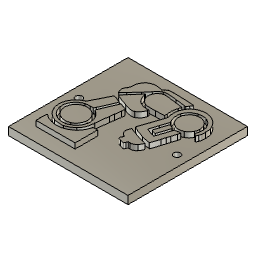
logo positive (Autodesk Fusion 360 design; units mm, degrees)
Autodesk Fusion 360 part; units mm, degrees
sketch "Sketch1" plane through (0, 0, 0) normal (0, 0, 1) x (1, 0, 0)
  line L0 (0, 0) -> (45, 0)
  line L1 (45, 0) -> (45, 45)
  line L2 (45, 45) -> (0, 45)
  line L3 (0, 45) -> (0, 0)
  dimension "d1" = 45
  dimension "d2" = 45
  constraint horizontal L0
  constraint vertical L1
  constraint horizontal L2
  constraint vertical L3
  constraint coincident L0.start L3.end
  measures "d1" distance of L0.start L0.end
  measures "d2" distance of L0.start L2.end
extrude "Extrude1" add sketch "Sketch1" along normal blind 3
sketch "Sketch2" plane through (0, 0, 3) normal (0, 0, 1) x (-1, 0, 0)
  line L0 (0, -45) -> (0, 0)
  line L1 (0, 0) -> (-45, 0)
  line L2 (-45, 0) -> (-45, -45)
  line L3 (-45, -45) -> (0, -45)
  spline S0 degree 3 poles (-20.2484, -39.8736) (-20.0856, -39.7573) (-19.7484, -39.4783) (-19.481, -39.2225) knots 0 0 0 0 1 1 1 1
  line L4 (-19.481, -39.2225) -> (-19.0044, -38.7691)
  line L5 (-19.0044, -38.7691) -> (-18.0859, -38.9668)
  spline S1 degree 3 poles (-18.0859, -38.9668) (-16.8071, -39.2342) (-15.5166, -39.1528) (-14.6447, -38.7575) knots 0 0 0 0 1 1 1 1
  spline S2 degree 3 poles (-14.6447, -38.7575) (-13.0519, -38.0251) (-12.1218, -36.3975) (-12.1102, -34.3164) knots 0 0 0 0 1 1 1 1
  spline S3 degree 3 poles (-12.1102, -34.3164) (-12.0986, -33.8281) (-12.0288, -33.6072) (-11.6452, -33.0376) knots 0 0 0 0 1 1 1 1
  spline S4 degree 3 poles (-11.6452, -33.0376) (-11.1685, -32.3168) (-10.9825, -31.6076) (-11.1104, -30.9798) knots 0 0 0 0 1 1 1 1
  spline S5 degree 3 poles (-11.1104, -30.9798) (-11.1918, -30.5264) (-11.5289, -29.8288) (-11.6452, -29.8288) knots 0 0 0 0 1 1 1 1
  spline S6 degree 3 poles (-11.6452, -29.8288) (-11.7033, -29.8288) (-12.3892, -30.5147) (-13.1798, -31.3634) knots 0 0 0 0 1 1 1 1
  spline S7 degree 3 poles (-13.1798, -31.3634) (-13.9704, -32.2005) (-15.1795, -33.491) (-15.8654, -34.2234) knots 0 0 0 0 1 1 1 1
  spline S8 degree 3 poles (-15.8654, -34.2234) (-16.5629, -34.9558) (-17.4116, -35.9324) (-17.7488, -36.3975) knots 0 0 0 0 1 1 1 1
  spline S9 degree 3 poles (-17.7488, -36.3975) (-18.4463, -37.3392) (-19.2369, -38.0716) (-19.8763, -38.3855) knots 0 0 0 0 1 1 1 1
  spline S10 degree 3 poles (-19.8763, -38.3855) (-20.5739, -38.7226) (-21.6086, -38.711) (-24.7825, -38.3274) knots 0 0 0 0 1 1 1 1
  spline S11 degree 3 poles (-24.7825, -38.3274) (-26.4101, -38.1297) (-28.0144, -37.9321) (-28.3283, -37.8972) knots 0 0 0 0 1 1 1 1
  line L6 (-28.3283, -37.8972) -> (-28.9096, -37.8391)
  line L7 (-28.9096, -37.8391) -> (-29.5142, -38.7459)
  spline S12 degree 3 poles (-29.5142, -38.7459) (-30.0374, -39.5248) (-30.0955, -39.6643) (-29.9211, -39.7225) knots 0 0 0 0 1 1 1 1
  spline S13 degree 3 poles (-29.9211, -39.7225) (-29.6421, -39.8271) (-24.3639, -40.0596) (-22.2713, -40.0596) knots 0 0 0 0 1 1 1 1
  spline S14 degree 3 poles (-22.2713, -40.0596) (-20.8529, -40.0596) (-20.4809, -40.0247) (-20.2484, -39.8736) knots 0 0 0 0 1 1 1 1
  spline S15 degree 3 poles (-33.0368, -39.3272) (-31.9789, -39.0133) (-30.8628, -38.3506) (-30.3164, -37.7228) knots 0 0 0 0 1 1 1 1
  spline S16 degree 3 poles (-30.3164, -37.7228) (-29.7816, -37.0834) (-29.1305, -35.8278) (-28.9096, -34.9907) knots 0 0 0 0 1 1 1 1
  spline S17 degree 3 poles (-28.9096, -34.9907) (-28.712, -34.235) (-28.6888, -32.712) (-28.8631, -31.9215) knots 0 0 0 0 1 1 1 1
  spline S18 degree 3 poles (-28.8631, -31.9215) (-29.084, -30.91) (-29.1073, -30.5264) (-28.991, -30.3869) knots 0 0 0 0 1 1 1 1
  spline S19 degree 3 poles (-28.991, -30.3869) (-28.9329, -30.3055) (-28.8166, -30.0497) (-28.7585, -29.8288) knots 0 0 0 0 1 1 1 1
  spline S20 degree 3 poles (-28.7585, -29.8288) (-28.6888, -29.6079) (-28.1075, -27.8757) (-27.4564, -25.9923) knots 0 0 0 0 1 1 1 1
  spline S21 degree 3 poles (-27.4564, -25.9923) (-26.2008, -22.3534) (-26.0264, -21.7953) (-26.0846, -21.7604) knots 0 0 0 0 1 1 1 1
  spline S22 degree 3 poles (-26.0846, -21.7604) (-26.724, -21.2954) (-28.8864, -20.4002) (-30.4908, -19.9352) knots 0 0 0 0 1 1 1 1
  spline S23 degree 3 poles (-30.4908, -19.9352) (-31.8742, -19.5399) (-33.56, -19.2028) (-33.7576, -19.2841) knots 0 0 0 0 1 1 1 1
  spline S24 degree 3 poles (-33.7576, -19.2841) (-33.9088, -19.3423) (-34.1413, -19.9701) (-34.897, -22.5045) knots 0 0 0 0 1 1 1 1
  spline S25 degree 3 poles (-34.897, -22.5045) (-35.0946, -23.1788) (-35.3039, -23.8531) (-35.362, -24.0159) knots 0 0 0 0 1 1 1 1
  spline S26 degree 3 poles (-35.362, -24.0159) (-35.4201, -24.1786) (-35.5945, -24.7832) (-35.7689, -25.3529) knots 0 0 0 0 1 1 1 1
  spline S27 degree 3 poles (-35.7689, -25.3529) (-35.9433, -25.9341) (-36.2107, -26.8061) (-36.3735, -27.3176) knots 0 0 0 0 1 1 1 1
  spline S28 degree 3 poles (-36.3735, -27.3176) (-36.5246, -27.8175) (-36.6292, -28.2477) (-36.606, -28.2826) knots 0 0 0 0 1 1 1 1
  spline S29 degree 3 poles (-36.606, -28.2826) (-36.5711, -28.3058) (-36.0828, -28.271) (-35.5015, -28.1896) knots 0 0 0 0 1 1 1 1
  line L8 (-35.5015, -28.1896) -> (-34.4552, -28.0617)
  line L9 (-34.4552, -28.0617) -> (-33.5135, -25.1668)
  spline S30 degree 3 poles (-33.5135, -25.1668) (-32.9903, -23.5857) (-32.5253, -22.2604) (-32.4788, -22.2255) knots 0 0 0 0 1 1 1 1
  spline S31 degree 3 poles (-32.4788, -22.2255) (-32.3625, -22.1557) (-29.3282, -23.1439) (-29.177, -23.2951) knots 0 0 0 0 1 1 1 1
  spline S32 degree 3 poles (-29.177, -23.2951) (-29.0957, -23.3764) (-29.4444, -24.5855) (-30.1187, -26.6084) knots 0 0 0 0 1 1 1 1
  line L10 (-30.1187, -26.6084) -> (-31.1767, -29.8056)
  line L11 (-31.1767, -29.8056) -> (-30.886, -30.3055)
  spline S33 degree 3 poles (-30.886, -30.3055) (-30.1769, -31.5495) (-29.9327, -33.305) (-30.3048, -34.5489) knots 0 0 0 0 1 1 1 1
  spline S34 degree 3 poles (-30.3048, -34.5489) (-30.7117, -35.9208) (-32.1533, -37.2926) (-33.6414, -37.7461) knots 0 0 0 0 1 1 1 1
  spline S35 degree 3 poles (-33.6414, -37.7461) (-34.5133, -38.0135) (-35.7805, -38.0135) (-36.6641, -37.7461) knots 0 0 0 0 1 1 1 1
  spline S36 degree 3 poles (-36.6641, -37.7461) (-37.8267, -37.3857) (-39.0707, -36.1766) (-39.5822, -34.9093) knots 0 0 0 0 1 1 1 1
  spline S37 degree 3 poles (-39.5822, -34.9093) (-39.8961, -34.142) (-39.9194, -32.3633) (-39.6171, -31.5843) knots 0 0 0 0 1 1 1 1
  spline S38 degree 3 poles (-39.6171, -31.5843) (-39.3264, -30.8054) (-39.373, -30.5961) (-39.838, -30.3752) knots 0 0 0 0 1 1 1 1
  spline S39 degree 3 poles (-39.838, -30.3752) (-40.0705, -30.2706) (-40.2681, -30.1776) (-40.2914, -30.1776) knots 0 0 0 0 1 1 1 1
  spline S40 degree 3 poles (-40.2914, -30.1776) (-40.3146, -30.1776) (-40.489, -30.5264) (-40.6634, -30.9682) knots 0 0 0 0 1 1 1 1
  spline S41 degree 3 poles (-40.6634, -30.9682) (-40.9773, -31.689) (-41.0006, -31.8517) (-40.989, -33.2003) knots 0 0 0 0 1 1 1 1
  spline S42 degree 3 poles (-40.989, -33.2003) (-40.9773, -34.4443) (-40.9308, -34.7698) (-40.6983, -35.4093) knots 0 0 0 0 1 1 1 1
  spline S43 degree 3 poles (-40.6983, -35.4093) (-39.5125, -38.5715) (-36.2107, -40.2573) (-33.0368, -39.3272) knots 0 0 0 0 1 1 1 1
  spline S44 degree 3 poles (-20.6088, -37.5949) (-20.0042, -37.4322) (-19.2485, -36.8625) (-18.8649, -36.2928) knots 0 0 0 0 1 1 1 1
  spline S45 degree 3 poles (-18.8649, -36.2928) (-17.6093, -34.4676) (-18.5045, -31.8168) (-20.6669, -30.9914) knots 0 0 0 0 1 1 1 1
  spline S46 degree 3 poles (-20.6669, -30.9914) (-21.3412, -30.7356) (-21.4226, -30.7356) (-24.5383, -30.8054) knots 0 0 0 0 1 1 1 1
  spline S47 degree 3 poles (-24.5383, -30.8054) (-26.2938, -30.8403) (-27.7819, -30.9217) (-27.8401, -30.9798) knots 0 0 0 0 1 1 1 1
  spline S48 degree 3 poles (-27.8401, -30.9798) (-27.8982, -31.0379) (-27.8866, -31.4448) (-27.7936, -31.968) knots 0 0 0 0 1 1 1 1
  spline S49 degree 3 poles (-27.7936, -31.968) (-27.6075, -33.1771) (-27.7238, -34.6303) (-28.1075, -35.8394) knots 0 0 0 0 1 1 1 1
  spline S50 degree 3 poles (-28.1075, -35.8394) (-28.2818, -36.3742) (-28.3981, -36.8276) (-28.3749, -36.8509) knots 0 0 0 0 1 1 1 1
  spline S51 degree 3 poles (-28.3749, -36.8509) (-28.2935, -36.9322) (-21.8411, -37.7344) (-21.4109, -37.7228) knots 0 0 0 0 1 1 1 1
  spline S52 degree 3 poles (-21.4109, -37.7228) (-21.19, -37.7228) (-20.8296, -37.6647) (-20.6088, -37.5949) knots 0 0 0 0 1 1 1 1
  spline S53 degree 3 poles (-34.1297, -36.9322) (-33.0136, -36.6648) (-31.9905, -35.851) (-31.4325, -34.7698) knots 0 0 0 0 1 1 1 1
  spline S54 degree 3 poles (-31.4325, -34.7698) (-31.1534, -34.2583) (-31.1186, -34.0606) (-31.1186, -33.0259) knots 0 0 0 0 1 1 1 1
  spline S55 degree 3 poles (-31.1186, -33.0259) (-31.1186, -31.9796) (-31.1534, -31.8052) (-31.4441, -31.2472) knots 0 0 0 0 1 1 1 1
  spline S56 degree 3 poles (-31.4441, -31.2472) (-32.4672, -29.3057) (-34.7458, -28.5383) (-36.699, -29.48) knots 0 0 0 0 1 1 1 1
  spline S57 degree 3 poles (-36.699, -29.48) (-37.3849, -29.8172) (-38.1987, -30.6543) (-38.5824, -31.4332) knots 0 0 0 0 1 1 1 1
  spline S58 degree 3 poles (-38.5824, -31.4332) (-38.8614, -32.0145) (-38.9079, -32.2354) (-38.9079, -33.1422) knots 0 0 0 0 1 1 1 1
  spline S59 degree 3 poles (-38.9079, -33.1422) (-38.9079, -34.0723) (-38.873, -34.2699) (-38.5591, -34.8628) knots 0 0 0 0 1 1 1 1
  spline S60 degree 3 poles (-38.5591, -34.8628) (-37.7453, -36.4788) (-35.8736, -37.3392) (-34.1297, -36.9322) knots 0 0 0 0 1 1 1 1
  spline S61 degree 3 poles (-16.5281, -33.6189) (-16.1793, -33.212) (-15.2957, -32.2005) (-14.5633, -31.3867) knots 0 0 0 0 1 1 1 1
  spline S62 degree 3 poles (-14.5633, -31.3867) (-12.8427, -29.4335) (-12.5404, -29.0266) (-12.7031, -28.829) knots 0 0 0 0 1 1 1 1
  spline S63 degree 3 poles (-12.7031, -28.829) (-12.8659, -28.6314) (-14.6912, -27.9222) (-16.9931, -27.1549) knots 0 0 0 0 1 1 1 1
  spline S64 degree 3 poles (-16.9931, -27.1549) (-19.1904, -26.4224) (-20.1088, -26.3062) (-20.8529, -26.6782) knots 0 0 0 0 1 1 1 1
  spline S65 degree 3 poles (-20.8529, -26.6782) (-21.876, -27.1665) (-22.7712, -28.3291) (-22.9688, -29.4103) knots 0 0 0 0 1 1 1 1
  line L12 (-22.9688, -29.4103) -> (-23.0502, -29.8637)
  line L13 (-23.0502, -29.8637) -> (-22.3875, -29.7939)
  spline S66 degree 3 poles (-22.3875, -29.7939) (-21.0505, -29.6544) (-19.7368, -30.1311) (-18.7254, -31.1193) knots 0 0 0 0 1 1 1 1
  spline S67 degree 3 poles (-18.7254, -31.1193) (-18.0627, -31.7703) (-17.4814, -32.9097) (-17.3768, -33.7933) knots 0 0 0 0 1 1 1 1
  spline S68 degree 3 poles (-17.3768, -33.7933) (-17.3419, -34.1072) (-17.2721, -34.3629) (-17.2372, -34.3513) knots 0 0 0 0 1 1 1 1
  spline S69 degree 3 poles (-17.2372, -34.3513) (-17.2024, -34.3513) (-16.8768, -34.0141) (-16.5281, -33.6189) knots 0 0 0 0 1 1 1 1
  spline S70 degree 3 poles (-31.8394, -28.9336) (-31.665, -28.643) (-30.235, -24.0856) (-30.2699, -23.9345) knots 0 0 0 0 1 1 1 1
  spline S71 degree 3 poles (-30.2699, -23.9345) (-30.3048, -23.7485) (-31.8161, -23.2253) (-31.944, -23.3532) knots 0 0 0 0 1 1 1 1
  spline S72 degree 3 poles (-31.944, -23.3532) (-32.0138, -23.423) (-33.2694, -27.3641) (-33.4321, -28.0036) knots 0 0 0 0 1 1 1 1
  spline S73 degree 3 poles (-33.4321, -28.0036) (-33.4902, -28.271) (-33.467, -28.3407) (-33.2112, -28.4337) knots 0 0 0 0 1 1 1 1
  spline S74 degree 3 poles (-33.2112, -28.4337) (-33.0601, -28.4918) (-32.6997, -28.6546) (-32.4323, -28.7825) knots 0 0 0 0 1 1 1 1
  spline S75 degree 3 poles (-32.4323, -28.7825) (-31.8742, -29.0499) (-31.9091, -29.0383) (-31.8394, -28.9336) knots 0 0 0 0 1 1 1 1
  spline S76 degree 3 poles (-11.901, -27.8175) (-11.8312, -27.7362) (-11.0174, -26.1434) (-10.0873, -24.2833) knots 0 0 0 0 1 1 1 1
  line L14 (-10.0873, -24.2833) -> (-8.3899, -20.8769)
  line L15 (-8.3899, -20.8769) -> (-7.5994, -20.5049)
  spline S77 degree 3 poles (-7.5994, -20.5049) (-6.5065, -19.9701) (-5.3207, -18.7726) (-4.751, -17.6216) knots 0 0 0 0 1 1 1 1
  spline S78 degree 3 poles (-4.751, -17.6216) (-4.007, -16.1103) (-3.914, -14.3896) (-4.4953, -12.7155) knots 0 0 0 0 1 1 1 1
  spline S79 degree 3 poles (-4.4953, -12.7155) (-5.0998, -10.9832) (-6.5879, -9.5533) (-8.4597, -8.8906) knots 0 0 0 0 1 1 1 1
  spline S80 degree 3 poles (-8.4597, -8.8906) (-9.3433, -8.5883) (-11.1453, -8.472) (-12.0056, -8.6697) knots 0 0 0 0 1 1 1 1
  spline S81 degree 3 poles (-12.0056, -8.6697) (-13.1914, -8.9371) (-14.3075, -9.5649) (-15.2027, -10.4601) knots 0 0 0 0 1 1 1 1
  spline S82 degree 3 poles (-15.2027, -10.4601) (-16.5164, -11.7738) (-16.9931, -12.948) (-17.1675, -15.3546) knots 0 0 0 0 1 1 1 1
  spline S83 degree 3 poles (-17.1675, -15.3546) (-17.2256, -16.2498) (-17.4814, -18.3889) (-17.7488, -20.2956) knots 0 0 0 0 1 1 1 1
  spline S84 degree 3 poles (-17.7488, -20.2956) (-17.7837, -20.5862) (-17.8883, -21.3419) (-17.9697, -21.9813) knots 0 0 0 0 1 1 1 1
  spline S85 degree 3 poles (-17.9697, -21.9813) (-18.0627, -22.6208) (-18.2022, -23.6438) (-18.2836, -24.26) knots 0 0 0 0 1 1 1 1
  spline S86 degree 3 poles (-18.2836, -24.26) (-18.365, -24.8646) (-18.3998, -25.4459) (-18.365, -25.5505) knots 0 0 0 0 1 1 1 1
  spline S87 degree 3 poles (-18.365, -25.5505) (-18.3185, -25.6551) (-17.772, -25.8993) (-17.0512, -26.1434) knots 0 0 0 0 1 1 1 1
  line L16 (-17.0512, -26.1434) -> (-15.8189, -26.5619)
  line L17 (-15.8189, -26.5619) -> (-15.6561, -26.1899)
  spline S88 degree 3 poles (-15.6561, -26.1899) (-15.4004, -25.6202) (-14.0169, -22.3766) (-13.4239, -20.935) knots 0 0 0 0 1 1 1 1
  line L18 (-13.4239, -20.935) -> (-12.8892, -19.6678)
  line L19 (-12.8892, -19.6678) -> (-13.1682, -19.4818)
  spline S89 degree 3 poles (-13.1682, -19.4818) (-15.3306, -18.0634) (-16.2258, -16.2033) (-15.8421, -13.9595) knots 0 0 0 0 1 1 1 1
  spline S90 degree 3 poles (-15.8421, -13.9595) (-15.4817, -11.8901) (-13.8192, -10.1694) (-11.7847, -9.7276) knots 0 0 0 0 1 1 1 1
  spline S91 degree 3 poles (-11.7847, -9.7276) (-8.7387, -9.0882) (-5.716, -11.1344) (-5.2509, -14.1687) knots 0 0 0 0 1 1 1 1
  spline S92 degree 3 poles (-5.2509, -14.1687) (-4.8673, -16.6799) (-6.46, -19.1446) (-8.9712, -19.8771) knots 0 0 0 0 1 1 1 1
  spline S93 degree 3 poles (-8.9712, -19.8771) (-9.413, -20.0166) (-9.9711, -20.0631) (-10.7732, -20.0514) knots 0 0 0 0 1 1 1 1
  line L20 (-10.7732, -20.0514) -> (-11.9358, -20.0166)
  line L21 (-11.9358, -20.0166) -> (-12.3079, -20.7722)
  spline S94 degree 3 poles (-12.3079, -20.7722) (-12.7496, -21.6558) (-14.9004, -26.6317) (-14.9004, -26.7828) knots 0 0 0 0 1 1 1 1
  spline S95 degree 3 poles (-14.9004, -26.7828) (-14.9004, -26.8293) (-14.5168, -27.0154) (-14.0634, -27.1781) knots 0 0 0 0 1 1 1 1
  spline S96 degree 3 poles (-14.0634, -27.1781) (-13.5983, -27.3409) (-12.9473, -27.585) (-12.6101, -27.7129) knots 0 0 0 0 1 1 1 1
  spline S97 degree 3 poles (-12.6101, -27.7129) (-12.1567, -27.8989) (-11.9823, -27.9222) (-11.901, -27.8175) knots 0 0 0 0 1 1 1 1
  spline S98 degree 3 poles (-25.7707, -20.3886) (-25.5498, -19.7957) (-25.3637, -19.0167) (-25.3637, -18.6912) knots 0 0 0 0 1 1 1 1
  spline S99 degree 3 poles (-25.3637, -18.6912) (-25.3637, -18.0518) (-25.8753, -17.1915) (-26.445, -16.9124) knots 0 0 0 0 1 1 1 1
  spline S100 degree 3 poles (-26.445, -16.9124) (-26.7123, -16.7729) (-26.9449, -16.6451) (-26.9681, -16.6334) knots 0 0 0 0 1 1 1 1
  spline S101 degree 3 poles (-26.9681, -16.6334) (-26.9797, -16.6218) (-26.8984, -16.3312) (-26.7589, -16.0056) knots 0 0 0 0 1 1 1 1
  spline S102 degree 3 poles (-26.7589, -16.0056) (-26.3752, -15.0291) (-26.3984, -15.0058) (-27.4913, -14.6687) knots 0 0 0 0 1 1 1 1
  spline S103 degree 3 poles (-27.4913, -14.6687) (-29.0027, -14.2036) (-28.9794, -14.2036) (-29.2817, -14.9477) knots 0 0 0 0 1 1 1 1
  line L22 (-29.2817, -14.9477) -> (-29.5374, -15.5871)
  line L23 (-29.5374, -15.5871) -> (-30.1769, -15.5522)
  spline S104 degree 3 poles (-30.1769, -15.5522) (-31.0372, -15.5057) (-31.7115, -15.808) (-32.2812, -16.4939) knots 0 0 0 0 1 1 1 1
  spline S105 degree 3 poles (-32.2812, -16.4939) (-32.6532, -16.9357) (-33.1531, -17.9239) (-33.1531, -18.2146) knots 0 0 0 0 1 1 1 1
  spline S106 degree 3 poles (-33.1531, -18.2146) (-33.1531, -18.2611) (-32.8043, -18.3541) (-32.3742, -18.4354) knots 0 0 0 0 1 1 1 1
  spline S107 degree 3 poles (-32.3742, -18.4354) (-31.3627, -18.6098) (-28.5027, -19.4934) (-27.096, -20.0747) knots 0 0 0 0 1 1 1 1
  spline S108 degree 3 poles (-27.096, -20.0747) (-25.852, -20.5862) (-25.8404, -20.5862) (-25.7707, -20.3886) knots 0 0 0 0 1 1 1 1
  spline S109 degree 3 poles (-9.32, -18.9586) (-7.3901, -18.4238) (-6.0183, -16.4242) (-6.2391, -14.4594) knots 0 0 0 0 1 1 1 1
  spline S110 degree 3 poles (-6.2391, -14.4594) (-6.3438, -13.5409) (-6.9716, -12.297) (-7.611, -11.7389) knots 0 0 0 0 1 1 1 1
  spline S111 degree 3 poles (-7.611, -11.7389) (-8.9131, -10.5996) (-10.936, -10.2857) (-12.4823, -10.9716) knots 0 0 0 0 1 1 1 1
  spline S112 degree 3 poles (-12.4823, -10.9716) (-15.1097, -12.1226) (-15.7259, -15.7615) (-13.6565, -17.8309) knots 0 0 0 0 1 1 1 1
  spline S113 degree 3 poles (-13.6565, -17.8309) (-12.5288, -18.9586) (-10.8779, -19.3888) (-9.32, -18.9586) knots 0 0 0 0 1 1 1 1
  spline S114 degree 3 poles (-18.2371, -13.5874) (-18.2022, -13.5293) (-18.1441, -13.3084) (-18.0976, -13.0875) knots 0 0 0 0 1 1 1 1
  spline S115 degree 3 poles (-18.0976, -13.0875) (-17.9464, -12.3435) (-17.1326, -10.8205) (-16.5048, -10.1113) knots 0 0 0 0 1 1 1 1
  spline S116 degree 3 poles (-16.5048, -10.1113) (-13.7844, -7.0188) (-9.4363, -6.5189) (-5.9485, -8.8906) knots 0 0 0 0 1 1 1 1
  line L24 (-5.9485, -8.8906) -> (-5.2858, -9.344)
  line L25 (-5.2858, -9.344) -> (-5.2044, -8.7511)
  spline S117 degree 3 poles (-5.2044, -8.7511) (-5.1696, -8.4139) (-5.1347, -7.4838) (-5.1347, -6.67) knots 0 0 0 0 1 1 1 1
  line L26 (-5.1347, -6.67) -> (-5.1347, -5.1819)
  line L27 (-5.1347, -5.1819) -> (-12.5171, -5.1819)
  line L28 (-12.5171, -5.1819) -> (-19.8996, -5.1819)
  line L29 (-19.8996, -5.1819) -> (-19.8996, -9.4254)
  line L30 (-19.8996, -9.4254) -> (-19.8996, -13.6688)
  line L31 (-19.8996, -13.6688) -> (-19.0974, -13.6688)
  spline S118 degree 3 poles (-19.0974, -13.6688) (-18.644, -13.6688) (-18.2603, -13.6339) (-18.2371, -13.5874) knots 0 0 0 0 1 1 1 1
extrude "Extrude2" add sketch "Sketch2" along normal blind 2 contours S0 L4 L5 S1 S2 S3 S4 S5 S6 S7 S8 S9 S10 S11 L6 L7 S12 S13 S14 | S15 S16 S17 S18 S19 S20 S21 S22 S23 S24 S25 S26 S27 S28 S29 L8 L9 S30 S31 S32 L10 L11 S33 S34 S35 S36 S37 S38 S39 S40 S41 S42 S43 | S44 S45 S46 S47 S48 S49 S50 S51 S52 | S53 S54 S55 S56 S57 S58 S59 S60 | S61 S62 S63 S64 S65 L12 L13 S66 S67 S68 S69 | S70 S71 S72 S73 S74 S75 | S76 L14 L15 S77 S78 S79 S80 S81 S82 S83 S84 S85 S86 S87 L16 L17 S88 L18 L19 S89 S90 S91 S92 S93 L20 L21 S94 S95 S96 S97 | S98 S99 S100 S101 S102 S103 L22 L23 S104 S105 S106 S107 S108 | S109 S110 S111 S112 S113 | S114 S115 S116 L24 L25 S117 L26 L27 L28 L29 L30 L31 S118
sketch "Sketch3" plane through (0, 0, 3) normal (0, 0, 1) x (-1, 0, 0)
  line L0 (-19.0974, -13.6688) -> (-19.8996, -13.6688)
  line L1 (-19.8996, -13.6688) -> (-19.8996, -5.1819)
  line L2 (-19.8996, -5.1819) -> (-5.1347, -5.1819)
  line L3 (-5.1347, -5.1819) -> (-5.1347, -6.67)
  spline S0 degree 3 poles (-5.1347, -6.67) (-5.1347, -7.4838) (-5.1696, -8.4139) (-5.2044, -8.7511) knots -1 -1 -1 -1 0 0 0 0
  line L4 (-5.2044, -8.7511) -> (-5.2858, -9.344)
  line L5 (-5.2858, -9.344) -> (-5.9485, -8.8906)
  spline S1 degree 3 poles (-5.9485, -8.8906) (-9.4363, -6.5189) (-13.7844, -7.0188) (-16.5048, -10.1113) knots -1 -1 -1 -1 0 0 0 0
  spline S2 degree 3 poles (-16.5048, -10.1113) (-17.1326, -10.8205) (-17.9464, -12.3435) (-18.0976, -13.0875) knots -1 -1 -1 -1 0 0 0 0
  spline S3 degree 3 poles (-18.0976, -13.0875) (-18.1441, -13.3084) (-18.2022, -13.5293) (-18.2371, -13.5874) knots -1 -1 -1 -1 0 0 0 0
  spline S4 degree 3 poles (-18.2371, -13.5874) (-18.2603, -13.6339) (-18.644, -13.6688) (-19.0974, -13.6688) knots -1 -1 -1 -1 0 0 0 0
  spline S5 degree 3 poles (-32.4323, -28.7825) (-32.6997, -28.6546) (-33.0601, -28.4918) (-33.2112, -28.4337) knots -1 -1 -1 -1 0 0 0 0
  spline S6 degree 3 poles (-33.2112, -28.4337) (-33.467, -28.3407) (-33.4902, -28.271) (-33.4321, -28.0036) knots -1 -1 -1 -1 0 0 0 0
  spline S7 degree 3 poles (-33.4321, -28.0036) (-33.2694, -27.3641) (-32.0138, -23.423) (-31.944, -23.3532) knots -1 -1 -1 -1 0 0 0 0
  spline S8 degree 3 poles (-31.944, -23.3532) (-31.8161, -23.2253) (-30.3048, -23.7485) (-30.2699, -23.9345) knots -1 -1 -1 -1 0 0 0 0
  spline S9 degree 3 poles (-30.2699, -23.9345) (-30.235, -24.0856) (-31.665, -28.643) (-31.8394, -28.9336) knots -1 -1 -1 -1 0 0 0 0
  spline S10 degree 3 poles (-31.8394, -28.9336) (-31.9091, -29.0383) (-31.8742, -29.0499) (-32.4323, -28.7825) knots -1 -1 -1 -1 0 0 0 0
  spline S11 degree 3 poles (-22.2713, -40.0596) (-24.3639, -40.0596) (-29.6421, -39.8271) (-29.9211, -39.7225) knots -1 -1 -1 -1 0 0 0 0
  spline S12 degree 3 poles (-29.9211, -39.7225) (-30.0955, -39.6643) (-30.0374, -39.5248) (-29.5142, -38.7459) knots -1 -1 -1 -1 0 0 0 0
  line L6 (-29.5142, -38.7459) -> (-28.9096, -37.8391)
  line L7 (-28.9096, -37.8391) -> (-28.3283, -37.8972)
  spline S13 degree 3 poles (-28.3283, -37.8972) (-28.0144, -37.9321) (-26.4101, -38.1297) (-24.7825, -38.3274) knots -1 -1 -1 -1 0 0 0 0
  spline S14 degree 3 poles (-24.7825, -38.3274) (-21.6086, -38.711) (-20.5739, -38.7226) (-19.8763, -38.3855) knots -1 -1 -1 -1 0 0 0 0
  spline S15 degree 3 poles (-19.8763, -38.3855) (-19.2369, -38.0716) (-18.4463, -37.3392) (-17.7488, -36.3975) knots -1 -1 -1 -1 0 0 0 0
  spline S16 degree 3 poles (-17.7488, -36.3975) (-17.4116, -35.9324) (-16.5629, -34.9558) (-15.8654, -34.2234) knots -1 -1 -1 -1 0 0 0 0
  spline S17 degree 3 poles (-15.8654, -34.2234) (-15.1795, -33.491) (-13.9704, -32.2005) (-13.1798, -31.3634) knots -1 -1 -1 -1 0 0 0 0
  spline S18 degree 3 poles (-13.1798, -31.3634) (-12.3892, -30.5147) (-11.7033, -29.8288) (-11.6452, -29.8288) knots -1 -1 -1 -1 0 0 0 0
  spline S19 degree 3 poles (-11.6452, -29.8288) (-11.5289, -29.8288) (-11.1918, -30.5264) (-11.1104, -30.9798) knots -1 -1 -1 -1 0 0 0 0
  spline S20 degree 3 poles (-11.1104, -30.9798) (-10.9825, -31.6076) (-11.1685, -32.3168) (-11.6452, -33.0376) knots -1 -1 -1 -1 0 0 0 0
  spline S21 degree 3 poles (-11.6452, -33.0376) (-12.0288, -33.6072) (-12.0986, -33.8281) (-12.1102, -34.3164) knots -1 -1 -1 -1 0 0 0 0
  spline S22 degree 3 poles (-12.1102, -34.3164) (-12.1218, -36.3975) (-13.0519, -38.0251) (-14.6447, -38.7575) knots -1 -1 -1 -1 0 0 0 0
  spline S23 degree 3 poles (-14.6447, -38.7575) (-15.5166, -39.1528) (-16.8071, -39.2342) (-18.0859, -38.9668) knots -1 -1 -1 -1 0 0 0 0
  line L8 (-18.0859, -38.9668) -> (-19.0044, -38.7691)
  line L9 (-19.0044, -38.7691) -> (-19.481, -39.2225)
  spline S24 degree 3 poles (-19.481, -39.2225) (-19.7484, -39.4783) (-20.0856, -39.7573) (-20.2484, -39.8736) knots -1 -1 -1 -1 0 0 0 0
  spline S25 degree 3 poles (-20.2484, -39.8736) (-20.4809, -40.0247) (-20.8529, -40.0596) (-22.2713, -40.0596) knots -1 -1 -1 -1 0 0 0 0
  spline S26 degree 3 poles (-21.4109, -37.7228) (-21.8411, -37.7344) (-28.2935, -36.9322) (-28.3749, -36.8509) knots -1 -1 -1 -1 0 0 0 0
  spline S27 degree 3 poles (-28.3749, -36.8509) (-28.3981, -36.8276) (-28.2818, -36.3742) (-28.1075, -35.8394) knots -1 -1 -1 -1 0 0 0 0
  spline S28 degree 3 poles (-28.1075, -35.8394) (-27.7238, -34.6303) (-27.6075, -33.1771) (-27.7936, -31.968) knots -1 -1 -1 -1 0 0 0 0
  spline S29 degree 3 poles (-27.7936, -31.968) (-27.8866, -31.4448) (-27.8982, -31.0379) (-27.8401, -30.9798) knots -1 -1 -1 -1 0 0 0 0
  spline S30 degree 3 poles (-27.8401, -30.9798) (-27.7819, -30.9217) (-26.2938, -30.8403) (-24.5383, -30.8054) knots -1 -1 -1 -1 0 0 0 0
  spline S31 degree 3 poles (-24.5383, -30.8054) (-21.4226, -30.7356) (-21.3412, -30.7356) (-20.6669, -30.9914) knots -1 -1 -1 -1 0 0 0 0
  spline S32 degree 3 poles (-20.6669, -30.9914) (-18.5045, -31.8168) (-17.6093, -34.4676) (-18.8649, -36.2928) knots -1 -1 -1 -1 0 0 0 0
  spline S33 degree 3 poles (-18.8649, -36.2928) (-19.2485, -36.8625) (-20.0042, -37.4322) (-20.6088, -37.5949) knots -1 -1 -1 -1 0 0 0 0
  spline S34 degree 3 poles (-20.6088, -37.5949) (-20.8296, -37.6647) (-21.19, -37.7228) (-21.4109, -37.7228) knots -1 -1 -1 -1 0 0 0 0
  spline S35 degree 3 poles (-27.096, -20.0747) (-28.5027, -19.4934) (-31.3627, -18.6098) (-32.3742, -18.4354) knots -1 -1 -1 -1 0 0 0 0
  spline S36 degree 3 poles (-32.3742, -18.4354) (-32.8043, -18.3541) (-33.1531, -18.2611) (-33.1531, -18.2146) knots -1 -1 -1 -1 0 0 0 0
  spline S37 degree 3 poles (-33.1531, -18.2146) (-33.1531, -17.9239) (-32.6532, -16.9357) (-32.2812, -16.4939) knots -1 -1 -1 -1 0 0 0 0
  spline S38 degree 3 poles (-32.2812, -16.4939) (-31.7115, -15.808) (-31.0372, -15.5057) (-30.1769, -15.5522) knots -1 -1 -1 -1 0 0 0 0
  line L10 (-30.1769, -15.5522) -> (-29.5374, -15.5871)
  line L11 (-29.5374, -15.5871) -> (-29.2817, -14.9477)
  spline S39 degree 3 poles (-29.2817, -14.9477) (-28.9794, -14.2036) (-29.0027, -14.2036) (-27.4913, -14.6687) knots -1 -1 -1 -1 0 0 0 0
  spline S40 degree 3 poles (-27.4913, -14.6687) (-26.3984, -15.0058) (-26.3752, -15.0291) (-26.7589, -16.0056) knots -1 -1 -1 -1 0 0 0 0
  spline S41 degree 3 poles (-26.7589, -16.0056) (-26.8984, -16.3312) (-26.9797, -16.6218) (-26.9681, -16.6334) knots -1 -1 -1 -1 0 0 0 0
  spline S42 degree 3 poles (-26.9681, -16.6334) (-26.9449, -16.6451) (-26.7123, -16.7729) (-26.445, -16.9124) knots -1 -1 -1 -1 0 0 0 0
  spline S43 degree 3 poles (-26.445, -16.9124) (-25.8753, -17.1915) (-25.3637, -18.0518) (-25.3637, -18.6912) knots -1 -1 -1 -1 0 0 0 0
  spline S44 degree 3 poles (-25.3637, -18.6912) (-25.3637, -19.0167) (-25.5498, -19.7957) (-25.7707, -20.3886) knots -1 -1 -1 -1 0 0 0 0
  spline S45 degree 3 poles (-25.7707, -20.3886) (-25.8404, -20.5862) (-25.852, -20.5862) (-27.096, -20.0747) knots -1 -1 -1 -1 0 0 0 0
  spline S46 degree 3 poles (-13.6565, -17.8309) (-15.7259, -15.7615) (-15.1097, -12.1226) (-12.4823, -10.9716) knots -1 -1 -1 -1 0 0 0 0
  spline S47 degree 3 poles (-12.4823, -10.9716) (-10.936, -10.2857) (-8.9131, -10.5996) (-7.611, -11.7389) knots -1 -1 -1 -1 0 0 0 0
  spline S48 degree 3 poles (-7.611, -11.7389) (-6.9716, -12.297) (-6.3438, -13.5409) (-6.2391, -14.4594) knots -1 -1 -1 -1 0 0 0 0
  spline S49 degree 3 poles (-6.2391, -14.4594) (-6.0183, -16.4242) (-7.3901, -18.4238) (-9.32, -18.9586) knots -1 -1 -1 -1 0 0 0 0
  spline S50 degree 3 poles (-9.32, -18.9586) (-10.8779, -19.3888) (-12.5288, -18.9586) (-13.6565, -17.8309) knots -1 -1 -1 -1 0 0 0 0
  spline S51 degree 3 poles (-40.6983, -35.4093) (-40.9308, -34.7698) (-40.9773, -34.4443) (-40.989, -33.2003) knots -1 -1 -1 -1 0 0 0 0
  spline S52 degree 3 poles (-40.989, -33.2003) (-41.0006, -31.8517) (-40.9773, -31.689) (-40.6634, -30.9682) knots -1 -1 -1 -1 0 0 0 0
  spline S53 degree 3 poles (-40.6634, -30.9682) (-40.489, -30.5264) (-40.3146, -30.1776) (-40.2914, -30.1776) knots -1 -1 -1 -1 0 0 0 0
  spline S54 degree 3 poles (-40.2914, -30.1776) (-40.2681, -30.1776) (-40.0705, -30.2706) (-39.838, -30.3752) knots -1 -1 -1 -1 0 0 0 0
  spline S55 degree 3 poles (-39.838, -30.3752) (-39.373, -30.5961) (-39.3264, -30.8054) (-39.6171, -31.5843) knots -1 -1 -1 -1 0 0 0 0
  spline S56 degree 3 poles (-39.6171, -31.5843) (-39.9194, -32.3633) (-39.8961, -34.142) (-39.5822, -34.9093) knots -1 -1 -1 -1 0 0 0 0
  spline S57 degree 3 poles (-39.5822, -34.9093) (-39.0707, -36.1766) (-37.8267, -37.3857) (-36.6641, -37.7461) knots -1 -1 -1 -1 0 0 0 0
  spline S58 degree 3 poles (-36.6641, -37.7461) (-35.7805, -38.0135) (-34.5133, -38.0135) (-33.6414, -37.7461) knots -1 -1 -1 -1 0 0 0 0
  spline S59 degree 3 poles (-33.6414, -37.7461) (-32.1533, -37.2926) (-30.7117, -35.9208) (-30.3048, -34.5489) knots -1 -1 -1 -1 0 0 0 0
  spline S60 degree 3 poles (-30.3048, -34.5489) (-29.9327, -33.305) (-30.1769, -31.5495) (-30.886, -30.3055) knots -1 -1 -1 -1 0 0 0 0
  line L12 (-30.886, -30.3055) -> (-31.1767, -29.8056)
  line L13 (-31.1767, -29.8056) -> (-30.1187, -26.6084)
  spline S61 degree 3 poles (-30.1187, -26.6084) (-29.4444, -24.5855) (-29.0957, -23.3764) (-29.177, -23.2951) knots -1 -1 -1 -1 0 0 0 0
  spline S62 degree 3 poles (-29.177, -23.2951) (-29.3282, -23.1439) (-32.3625, -22.1557) (-32.4788, -22.2255) knots -1 -1 -1 -1 0 0 0 0
  spline S63 degree 3 poles (-32.4788, -22.2255) (-32.5253, -22.2604) (-32.9903, -23.5857) (-33.5135, -25.1668) knots -1 -1 -1 -1 0 0 0 0
  line L14 (-33.5135, -25.1668) -> (-34.4552, -28.0617)
  line L15 (-34.4552, -28.0617) -> (-35.5015, -28.1896)
  spline S64 degree 3 poles (-35.5015, -28.1896) (-36.0828, -28.271) (-36.5711, -28.3058) (-36.606, -28.2826) knots -1 -1 -1 -1 0 0 0 0
  spline S65 degree 3 poles (-36.606, -28.2826) (-36.6292, -28.2477) (-36.5246, -27.8175) (-36.3735, -27.3176) knots -1 -1 -1 -1 0 0 0 0
  spline S66 degree 3 poles (-36.3735, -27.3176) (-36.2107, -26.8061) (-35.9433, -25.9341) (-35.7689, -25.3529) knots -1 -1 -1 -1 0 0 0 0
  spline S67 degree 3 poles (-35.7689, -25.3529) (-35.5945, -24.7832) (-35.4201, -24.1786) (-35.362, -24.0159) knots -1 -1 -1 -1 0 0 0 0
  spline S68 degree 3 poles (-35.362, -24.0159) (-35.3039, -23.8531) (-35.0946, -23.1788) (-34.897, -22.5045) knots -1 -1 -1 -1 0 0 0 0
  spline S69 degree 3 poles (-34.897, -22.5045) (-34.1413, -19.9701) (-33.9088, -19.3423) (-33.7576, -19.2841) knots -1 -1 -1 -1 0 0 0 0
  spline S70 degree 3 poles (-33.7576, -19.2841) (-33.56, -19.2028) (-31.8742, -19.5399) (-30.4908, -19.9352) knots -1 -1 -1 -1 0 0 0 0
  spline S71 degree 3 poles (-30.4908, -19.9352) (-28.8864, -20.4002) (-26.724, -21.2954) (-26.0846, -21.7604) knots -1 -1 -1 -1 0 0 0 0
  spline S72 degree 3 poles (-26.0846, -21.7604) (-26.0264, -21.7953) (-26.2008, -22.3534) (-27.4564, -25.9923) knots -1 -1 -1 -1 0 0 0 0
  spline S73 degree 3 poles (-27.4564, -25.9923) (-28.1075, -27.8757) (-28.6888, -29.6079) (-28.7585, -29.8288) knots -1 -1 -1 -1 0 0 0 0
  spline S74 degree 3 poles (-28.7585, -29.8288) (-28.8166, -30.0497) (-28.9329, -30.3055) (-28.991, -30.3869) knots -1 -1 -1 -1 0 0 0 0
  spline S75 degree 3 poles (-28.991, -30.3869) (-29.1073, -30.5264) (-29.084, -30.91) (-28.8631, -31.9215) knots -1 -1 -1 -1 0 0 0 0
  spline S76 degree 3 poles (-28.8631, -31.9215) (-28.6888, -32.712) (-28.712, -34.235) (-28.9096, -34.9907) knots -1 -1 -1 -1 0 0 0 0
  spline S77 degree 3 poles (-28.9096, -34.9907) (-29.1305, -35.8278) (-29.7816, -37.0834) (-30.3164, -37.7228) knots -1 -1 -1 -1 0 0 0 0
  spline S78 degree 3 poles (-30.3164, -37.7228) (-30.8628, -38.3506) (-31.9789, -39.0133) (-33.0368, -39.3272) knots -1 -1 -1 -1 0 0 0 0
  spline S79 degree 3 poles (-33.0368, -39.3272) (-36.2107, -40.2573) (-39.5125, -38.5715) (-40.6983, -35.4093) knots -1 -1 -1 -1 0 0 0 0
  spline S80 degree 3 poles (-17.2372, -34.3513) (-17.2721, -34.3629) (-17.3419, -34.1072) (-17.3768, -33.7933) knots -1 -1 -1 -1 0 0 0 0
  spline S81 degree 3 poles (-17.3768, -33.7933) (-17.4814, -32.9097) (-18.0627, -31.7703) (-18.7254, -31.1193) knots -1 -1 -1 -1 0 0 0 0
  spline S82 degree 3 poles (-18.7254, -31.1193) (-19.7368, -30.1311) (-21.0505, -29.6544) (-22.3875, -29.7939) knots -1 -1 -1 -1 0 0 0 0
  line L16 (-22.3875, -29.7939) -> (-23.0502, -29.8637)
  line L17 (-23.0502, -29.8637) -> (-22.9688, -29.4103)
  spline S83 degree 3 poles (-22.9688, -29.4103) (-22.7712, -28.3291) (-21.876, -27.1665) (-20.8529, -26.6782) knots -1 -1 -1 -1 0 0 0 0
  spline S84 degree 3 poles (-20.8529, -26.6782) (-20.1088, -26.3062) (-19.1904, -26.4224) (-16.9931, -27.1549) knots -1 -1 -1 -1 0 0 0 0
  spline S85 degree 3 poles (-16.9931, -27.1549) (-14.6912, -27.9222) (-12.8659, -28.6314) (-12.7031, -28.829) knots -1 -1 -1 -1 0 0 0 0
  spline S86 degree 3 poles (-12.7031, -28.829) (-12.5404, -29.0266) (-12.8427, -29.4335) (-14.5633, -31.3867) knots -1 -1 -1 -1 0 0 0 0
  spline S87 degree 3 poles (-14.5633, -31.3867) (-15.2957, -32.2005) (-16.1793, -33.212) (-16.5281, -33.6189) knots -1 -1 -1 -1 0 0 0 0
  spline S88 degree 3 poles (-16.5281, -33.6189) (-16.8768, -34.0141) (-17.2024, -34.3513) (-17.2372, -34.3513) knots -1 -1 -1 -1 0 0 0 0
  spline S89 degree 3 poles (-38.5591, -34.8628) (-38.873, -34.2699) (-38.9079, -34.0723) (-38.9079, -33.1422) knots -1 -1 -1 -1 0 0 0 0
  spline S90 degree 3 poles (-38.9079, -33.1422) (-38.9079, -32.2354) (-38.8614, -32.0145) (-38.5824, -31.4332) knots -1 -1 -1 -1 0 0 0 0
  spline S91 degree 3 poles (-38.5824, -31.4332) (-38.1987, -30.6543) (-37.3849, -29.8172) (-36.699, -29.48) knots -1 -1 -1 -1 0 0 0 0
  spline S92 degree 3 poles (-36.699, -29.48) (-34.7458, -28.5383) (-32.4672, -29.3057) (-31.4441, -31.2472) knots -1 -1 -1 -1 0 0 0 0
  spline S93 degree 3 poles (-31.4441, -31.2472) (-31.1534, -31.8052) (-31.1186, -31.9796) (-31.1186, -33.0259) knots -1 -1 -1 -1 0 0 0 0
  spline S94 degree 3 poles (-31.1186, -33.0259) (-31.1186, -34.0606) (-31.1534, -34.2583) (-31.4325, -34.7698) knots -1 -1 -1 -1 0 0 0 0
  spline S95 degree 3 poles (-31.4325, -34.7698) (-31.9905, -35.851) (-33.0136, -36.6648) (-34.1297, -36.9322) knots -1 -1 -1 -1 0 0 0 0
  spline S96 degree 3 poles (-34.1297, -36.9322) (-35.8736, -37.3392) (-37.7453, -36.4788) (-38.5591, -34.8628) knots -1 -1 -1 -1 0 0 0 0
  spline S97 degree 3 poles (-12.6101, -27.7129) (-12.9473, -27.585) (-13.5983, -27.3409) (-14.0634, -27.1781) knots -1 -1 -1 -1 0 0 0 0
  spline S98 degree 3 poles (-14.0634, -27.1781) (-14.5168, -27.0154) (-14.9004, -26.8293) (-14.9004, -26.7828) knots -1 -1 -1 -1 0 0 0 0
  spline S99 degree 3 poles (-14.9004, -26.7828) (-14.9004, -26.6317) (-12.7496, -21.6558) (-12.3079, -20.7722) knots -1 -1 -1 -1 0 0 0 0
  line L18 (-12.3079, -20.7722) -> (-11.9358, -20.0166)
  line L19 (-11.9358, -20.0166) -> (-10.7732, -20.0514)
  spline S100 degree 3 poles (-10.7732, -20.0514) (-9.9711, -20.0631) (-9.413, -20.0166) (-8.9712, -19.8771) knots -1 -1 -1 -1 0 0 0 0
  spline S101 degree 3 poles (-8.9712, -19.8771) (-6.46, -19.1446) (-4.8673, -16.6799) (-5.2509, -14.1687) knots -1 -1 -1 -1 0 0 0 0
  spline S102 degree 3 poles (-5.2509, -14.1687) (-5.716, -11.1344) (-8.7387, -9.0882) (-11.7847, -9.7276) knots -1 -1 -1 -1 0 0 0 0
  spline S103 degree 3 poles (-11.7847, -9.7276) (-13.8192, -10.1694) (-15.4817, -11.8901) (-15.8421, -13.9595) knots -1 -1 -1 -1 0 0 0 0
  spline S104 degree 3 poles (-15.8421, -13.9595) (-16.2258, -16.2033) (-15.3306, -18.0634) (-13.1682, -19.4818) knots -1 -1 -1 -1 0 0 0 0
  line L20 (-13.1682, -19.4818) -> (-12.8892, -19.6678)
  line L21 (-12.8892, -19.6678) -> (-13.4239, -20.935)
  spline S105 degree 3 poles (-13.4239, -20.935) (-14.0169, -22.3766) (-15.4004, -25.6202) (-15.6561, -26.1899) knots -1 -1 -1 -1 0 0 0 0
  line L22 (-15.6561, -26.1899) -> (-15.8189, -26.5619)
  line L23 (-15.8189, -26.5619) -> (-17.0512, -26.1434)
  spline S106 degree 3 poles (-17.0512, -26.1434) (-17.772, -25.8993) (-18.3185, -25.6551) (-18.365, -25.5505) knots -1 -1 -1 -1 0 0 0 0
  spline S107 degree 3 poles (-18.365, -25.5505) (-18.3998, -25.4459) (-18.365, -24.8646) (-18.2836, -24.26) knots -1 -1 -1 -1 0 0 0 0
  spline S108 degree 3 poles (-18.2836, -24.26) (-18.2022, -23.6438) (-18.0627, -22.6208) (-17.9697, -21.9813) knots -1 -1 -1 -1 0 0 0 0
  spline S109 degree 3 poles (-17.9697, -21.9813) (-17.8883, -21.3419) (-17.7837, -20.5862) (-17.7488, -20.2956) knots -1 -1 -1 -1 0 0 0 0
  spline S110 degree 3 poles (-17.7488, -20.2956) (-17.4814, -18.3889) (-17.2256, -16.2498) (-17.1675, -15.3546) knots -1 -1 -1 -1 0 0 0 0
  spline S111 degree 3 poles (-17.1675, -15.3546) (-16.9931, -12.948) (-16.5164, -11.7738) (-15.2027, -10.4601) knots -1 -1 -1 -1 0 0 0 0
  spline S112 degree 3 poles (-15.2027, -10.4601) (-14.3075, -9.5649) (-13.1914, -8.9371) (-12.0056, -8.6697) knots -1 -1 -1 -1 0 0 0 0
  spline S113 degree 3 poles (-12.0056, -8.6697) (-11.1453, -8.472) (-9.3433, -8.5883) (-8.4597, -8.8906) knots -1 -1 -1 -1 0 0 0 0
  spline S114 degree 3 poles (-8.4597, -8.8906) (-6.5879, -9.5533) (-5.0998, -10.9832) (-4.4953, -12.7155) knots -1 -1 -1 -1 0 0 0 0
  spline S115 degree 3 poles (-4.4953, -12.7155) (-3.914, -14.3896) (-4.007, -16.1103) (-4.751, -17.6216) knots -1 -1 -1 -1 0 0 0 0
  spline S116 degree 3 poles (-4.751, -17.6216) (-5.3207, -18.7726) (-6.5065, -19.9701) (-7.5994, -20.5049) knots -1 -1 -1 -1 0 0 0 0
  line L24 (-7.5994, -20.5049) -> (-8.3899, -20.8769)
  line L25 (-8.3899, -20.8769) -> (-10.0873, -24.2833)
  spline S117 degree 3 poles (-10.0873, -24.2833) (-11.0174, -26.1434) (-11.8312, -27.7362) (-11.901, -27.8175) knots -1 -1 -1 -1 0 0 0 0
  spline S118 degree 3 poles (-11.901, -27.8175) (-11.9823, -27.9222) (-12.1567, -27.8989) (-12.6101, -27.7129) knots -1 -1 -1 -1 0 0 0 0
  line L26 (0, -45) -> (0, 0)
  line L27 (0, 0) -> (-45, 0)
  line L28 (-45, 0) -> (-45, -45)
  line L29 (-45, -45) -> (0, -45)
  circle A0 centre (-4, -22.5) radius 1.25
  circle A1 centre (-41, -22.5) radius 1.25
  dimension "d8" = 2.5
  dimension "d10" = 2.5
  measures "d8" diameter of A0
  measures "d10" diameter of A1
extrude "Extrude3" cut sketch "Sketch3" against normal blind 2 contours A0 | A1
sketch "Sketch5" plane through (0, 0, 1) normal (0, 0, 1) x (-1, 0, 0)
  circle A0 centre (-41, -22.5) radius 1.25
  circle A1 centre (-41, -22.5) radius 0.75
  dimension "d17" = 1.5
  constraint concentric A0 A1
  measures "d17" diameter of A1
extrude "Extrude5" cut sketch "Sketch5" against normal blind 1 contours A1
sketch "Sketch6" plane through (0, 0, 1) normal (0, 0, 1) x (-1, 0, 0)
  circle A0 centre (-4, -22.5) radius 1.25
  circle A1 centre (-4, -22.5) radius 0.75
  dimension "d20" = 1.5
  constraint concentric A0 A1
  measures "d20" diameter of A1
extrude "Extrude6" cut sketch "Sketch6" against normal blind 1 contours A1
